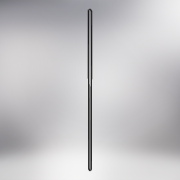
# Autodesk Inventor part: Courroie synchrone
Saved by Autodesk Inventor 2017 (Build 210142000, 142)
## iProperties
Created: 2016-07-28
Part Number: Courroie synchrone
Material: Caoutchouc
Document SubType Name: Modeling
Designer: FABLAB Frenchmakers
Density: 0.93 g/cm^3
Appearance: Caoutchouc - Noir
Project: 1420 Vauban 3D XL
Catalog Web Link: http://frenchmakers.com/
Mass: 4.75336 g
Surface Area: 187.408 cm^2
Volume: 5.11114 cm^3
Stock Number: 1420-20-03
CustomPartVersion: 1
Company: FABLAB Frenchmakers
Autodesk Inventor part; units mm, degrees
sketch "Chemin d'esquisse" plane through (0, 0, 0) normal (0, 0, 1) x (1, 0, 0)
  arc A0 (7.957682, -0.032157) -> (-7.957682, -0.032157) centre (0, 0) ccw
  arc A1 (-5.172493, -689.270902) -> (5.172493, -689.270902) centre (0, -689.25) ccw
  line L0 (-5.172493, -689.270902) -> (-7.957682, -0.032157)
  line L1 (7.957682, -0.032157) -> (5.172493, -689.270902)
  constraints: 4 end point, 2 point on circle, 1 centre point, 1 horizontal alignment, 2 other
ref_plane "Plan de section" through (-7.957682, -0.032157, 0) normal (0.0040409, -0.9999918, 0) x (0, 0, 1)
ref_plane "Plan de construction2" through (0, 0, 0) normal (-1, 0, 0) x (0, 0, 1)
ref_plane "Plan de construction3" through (0, -689.25, 0) normal (0.1434124, 0.989663, 0) x (0, 0, 1)
sketch "Section" plane through (-7.957682, -0.032157, 0) normal (0.0040409, -0.9999918, 0) x (0, 0, 1)
  line L0 (-3, 0.3) -> (3, 0.3)
  line L1 (3, 0.3) -> (3, -0.3)
  line L2 (3, -0.3) -> (-3, -0.3)
  line L3 (-3, -0.3) -> (-3, 0.3)
  line L4 (-3, 0) -> (3, 0) construction
  point P0 (0, 0)
  point P1 (0, 0)
  dimension "d0" = 6
  dimension "d4" = 0.3
  dimension "d5" = 0.3
  constraints: 10 end point, 3 midpoint, 2 parallel, 1 coincident, 1 horizontal, 1 perpendicular, 1 other
  measures "d0" distance between parallel lines of L1 L3
  measures "d4" distance between parallel lines of L2 L4
  measures "d5" distance between parallel lines of L4 L0
sweep "Courroie" add profiles "Section" path "Chemin d'esquisse"
equation "\"d0\" = da_B"
equation "\"d4\" = da_a"
equation "\"d5\" = da_a2"
equation "\"da_B\" = 6"
equation "\"da_pb\" = 2.5"
equation "\"da_L\" = 1419.76125"
equation "\"da_a\" = 0.3"
equation "\"da_S\" = 1.5"
equation "\"da_Beta\" = 20deg"
equation "\"da_Ht\" = 0.7"
equation "\"da_H\" = 1.3"
equation "\"da_a2\" = 0.3"
body "Solid1"
